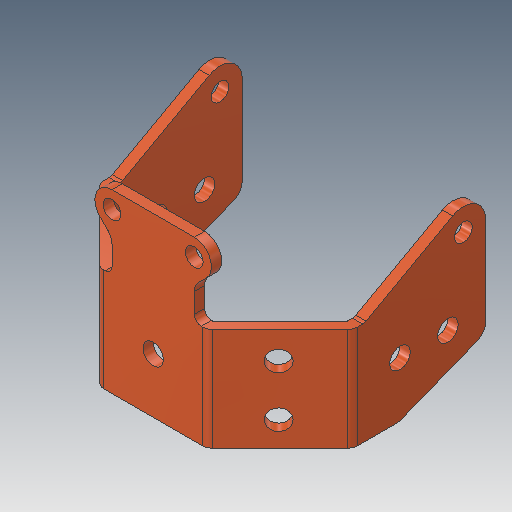
# Autodesk Inventor part: plate
Saved by Autodesk Inventor 2019.4 (Build 234330000, 330)
## iProperties
Created: 2018-07-18
Part Number: plate
Material: アルミニウム 6061
Document SubType Name: Modeling
Designer: student
Density: 2.7 g/cm^3
Appearance: 滑らか - 淡いオレンジ
Mass: 5.62142 g
Surface Area: 32.9137 cm^2
Volume: 2.08201 cm^3
Author: student
Autodesk Inventor part; units mm, degrees
ref_plane "YZ Plane" through (0, 0, 0) normal (1, 0, 0) x (0, 1, 0)
ref_plane "XZ Plane" through (0, 0, 0) normal (0, 1, 0) x (-1, 0, 0)
ref_plane "XY Plane" through (0, 0, 0) normal (0, 0, 1) x (1, 0, 0)
sketch "スケッチ1" plane through (0, 0, 0) normal (0, 1, 0) x (-1, 0, 0)
  line L0 (0, 0) -> (0, 28.5) construction
  line L1 (0, 30) -> (-7.1789, 30)
  line L2 (-8.2396, 29.5607) -> (-18.0607, 19.7396)
  line L3 (-18.5, 18.6789) -> (-18.5, 0)
  line L4 (-18.5, 0) -> (-17, 0)
  line L5 (-17, 0) -> (-17, 18.6789)
  line L6 (-17, 18.6789) -> (-7.1789, 28.5)
  line L7 (-7.1789, 28.5) -> (0, 28.5)
  line L8 (0, 28.5) -> (0, 30)
  line L9 (0, 0) -> (-17, 0) construction
  line L10 (0, 14.25) -> (-10.7145, 24.9645) construction
  arc A0 (-7.1789, 30) -> (-8.2396, 29.5607) centre (-7.1789, 28.5) ccw
  arc A1 (-18.0607, 19.7396) -> (-18.5, 18.6789) centre (-17, 18.6789) ccw
  dimension "d0" = 28.5
  dimension "d1" = 1.5
  dimension "d2" = 1.5
  dimension "d3" = 135
  dimension "d4" = 1.5
  dimension "d5" = 34
  dimension "d7" = 5
  dimension "d8" = 1.5
  constraints: 22 end point, 7 perpendicular, 4 point on circle, 4 tangent, 3 parallel, 2 centre point, 2 vertical, 1 equal radius, 1 horizontal, 1 midpoint, 1 point on line
  measures "d0" distance between parallel lines of L7 L4
  measures "d1" distance between parallel lines of L1 L7
  measures "d2" distance between parallel lines of L2 L6
  measures "d3" angle of L6 L7
  measures "d4" distance between parallel lines of L3 L5
  measures "d5" diameter of L5 L0
  measures "d7" distance from line of L10 L6.end
  measures "d8" radius of A0
extrude "押し出し1" add sketch "スケッチ1" against normal blind 15
sketch "スケッチ2" plane through (17, 0, 0) normal (-1, 0, 0) x (0, 0, 1)
  circle A0 centre (3.25, 4.25) radius 1.3
  arc A1 (4.8202, 7.0955) -> (0, 4.25) centre (3.25, 4.25) ccw
  line L0 (0, 4.25) -> (0, 0)
  line L1 (4.8202, 7.0955) -> (17.6789, 0)
  line L2 (18.6789, 0) -> (0, 0) construction
  line L3 (0, 0) -> (0, -15) construction
  line L4 (0, 0) -> (17.6789, 0)
  line L5 (18.6789, 0) -> (18.6789, -15) projected
  dimension "d11" = 2.6
  dimension "d12" = 4.25
  dimension "d13" = 3.25
  dimension "d14" = 1
  constraints: 6 end point, 2 centre point, 2 point on circle, 2 tangent, 1 collinear, 1 concentric, 1 vertical
  measures "d11" diameter of A0
  measures "d12" distance from line of L2 A0.centre
  measures "d13" radius of A1
  measures "d14" distance from line of L5 L1.end
extrude "押し出し2" add sketch "スケッチ2" against normal blind 1.5
sketch "スケッチ3" plane through (7.1789, 0, 28.5) normal (0, 0, -1) x (-1, 0, 0)
  circle A0 centre (1.1789, 8.25) radius 1.3
  line L0 (7.1789, 0) -> (0, 0) construction
  line L1 (7.1789, 0) -> (7.1789, 5.7754) construction
  arc A1 (1.1789, 10.75) -> (-0.5888, 6.4822) centre (1.1789, 8.25) ccw
  line L2 (-0.5888, 6.4822) -> (1.1789, 4.7145)
  line L3 (1.1789, 4.7145) -> (1.1789, 0)
  line L4 (1.1789, 10.75) -> (7.1789, 10.75)
  line L5 (7.1789, 10.75) -> (7.1789, 0)
  line L6 (1.1789, 0) -> (7.1789, 0)
  dimension "d17" = 8.25
  dimension "d18" = 12
  dimension "d19" = 2.6
  dimension "d20" = 2.5
  dimension "d21" = 45
  dimension "d22" = 12
  constraints: 12 end point, 2 centre point, 2 collinear, 2 point on circle, 2 tangent, 1 concentric, 1 horizontal, 1 perpendicular, 1 point on line, 1 vertical
  measures "d17" distance from line of L0 A0.centre
  measures "d18" diameter of A0.centre L1
  measures "d19" diameter of A0
  measures "d20" radius of A1
  measures "d21" angle of L3 L2
  measures "d22" diameter of L3 L1
extrude "押し出し3" add sketch "スケッチ3" against normal blind 1.5
sketch "スケッチ4" plane through (18.5, -15, 18.6789) normal (1, 0, 0) x (0, 0, -1)
  line L0 (6, 0) -> (18.6789, 5)
  line L1 (18.6789, 0) -> (18.6789, 19.25) construction
  line L2 (18.6789, 0) -> (18.6789, 5)
  line L3 (0, 0) -> (18.6789, 0) construction
  line L4 (18.6789, 0) -> (6, 0)
  line L5 (0, 15) -> (0, 0) construction
  circle A0 centre (13.1789, 8) radius 1.5
  circle A1 centre (6.1789, 8) radius 1.5
  arc A2 (14.2789, 7.4063) -> (14.2789, 8.5937) centre (13.1789, 8) ccw projected
  arc A3 (7.2789, 7.4063) -> (7.2789, 8.5937) centre (6.1789, 8) ccw projected
  dimension "d25" = 5
  dimension "d26" = 6
  dimension "d36" = 3
  constraints: 6 end point, 2 centre point, 2 collinear, 2 concentric, 1 equal radius, 1 point on line
  measures "d25" distance from line of L3 L0.end
  measures "d26" distance from line of L5 L0.start
  measures "d36" diameter of A0
extrude "押し出し4" cut sketch "スケッチ4" against normal blind 1.5
fillet "フィレット1" radius 2 3 edges at (17.75, -10, 0) (17.75, -15, 12.6789) (6, 4.7145, 29.25)
fillet "フィレット2" radius 1 2 edges at (17.75, 0, 17.6789) (6, 0, 29.25)
sketch "スケッチ5" plane through (8.2396, -15, 29.5607) normal (0.7071, 0, 0.7071) x (0.7071, 0, -0.7071)
  circle A0 centre (6.8, 11) radius 1.5
  circle A1 centre (6.8, 3.6) radius 1.5
  line L0 (0, 15) -> (13.8891, 15) projected
  line L1 (6.8, 90.0103) -> (6.8, -102.5616) construction
  point P0 (15.0763, 15)
  dimension "d31" = 7.4
  dimension "d32" = 3
  dimension "d33" = 4
  constraints: 2 centre point, 2 end point, 2 point on line, 1 equal radius, 1 vertical, 2 other
  measures "d31" distance of A1.centre A0.centre
  measures "d32" diameter of A0
  measures "d33" distance from line of L0 A0.centre
extrude "押し出し5" cut sketch "スケッチ5" against normal blind 1.5
mirror "ミラー3" about plane through (0, 0, 0) normal (1, 0, 0) of "押し出し1", "押し出し2", "押し出し3", "押し出し4", "フィレット1", "フィレット2", "押し出し5"
sketch "スケッチ7" plane through (7.1789, -15, 30) normal (0, 0, 1) x (1, 0, 0)
  circle A0 centre (-7.1789, 8) radius 1.5
  arc A1 (-7.8848, 9.0316) -> (-7.8848, 6.9684) centre (-7.1789, 8) ccw projected
  point P0 (-7.1789, 15)
  dimension "d37" = 3
  constraints: 1 centre point
  measures "d37" diameter of A0
extrude "押し出し6" cut sketch "スケッチ7" against normal blind 1.5
